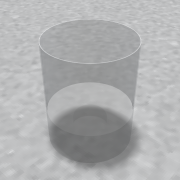
# Autodesk Inventor part: Visk
Saved by Autodesk Inventor 2013 (Build 170138000, 138)
## iProperties
Created: 2012-09-13
Part Number: Visk
Material: Generic
Document SubType Name: Modeling
Designer: bilal
Density: 1 g/cm^3
Mass: 297.655 g
Surface Area: 836.008 cm^2
Volume: 297.655 cm^3
Author: bilal
Autodesk Inventor part; units mm, degrees
ref_plane "YZ Plane" through (0, 0, 0) normal (1, 0, 0) x (0, 1, 0)
ref_plane "XZ Plane" through (0, 0, 0) normal (0, 1, 0) x (-1, 0, 0)
ref_plane "XY Plane" through (0, 0, 0) normal (0, 0, 1) x (1, 0, 0)
sketch "Sketch1" plane through (0, 0, 0) normal (0, 0, 1) x (1, 0, 0)
  line L0 (0, 0) -> (50, 0)
  line L1 (50, 0) -> (50, 20)
  line L2 (0, 0) -> (0, 125)
  line L3 (0, 125) -> (50, 125)
  line L4 (50, 125) -> (50, 20)
  dimension "d15" = 125
  constraints: 10 end point, 2 perpendicular
  measures "d15" distance of L0.start L2.end
revolve "Revolution1" add sketch "Sketch1" angle 360 about axis through (0, 0, 0) along (0, 1, 0)
shell "Shell1" thickness 1 removed faces 1 at (-6.8644, 125, 10.9394)
sketch "Sketch2" plane through (0, 1, 0) normal (0, 1, 0) x (1, 0, 0)
  circle A0 centre (0, 0) radius 49 projected
  circle A1 centre (0, 0) radius 49 projected
extrude "Extrusion1" add sketch "Sketch2" along normal blind 39
fillet "Fillet1" radius 0.5 3 edges at (-50, 125, 0) (-49, 125, 0) (-50, 0, 0)
sketch "Sketch3" plane through (0, 0, 0) normal (0, -1, 0) x (1, 0, 0)
  circle A0 centre (0, 0) radius 49.5 projected
  circle A1 centre (0, 0) radius 20
  constraints: 1 centre point, 1 coincident
extrude "Extrusion2" cut sketch "Sketch3" against normal blind 29 contours A1
fillet "Fillet2" radius 15 1 edges at (-20, 0, 0)
fillet "Fillet3" radius 5 1 edges at (-20, 29, 0)
body "Solid1"
